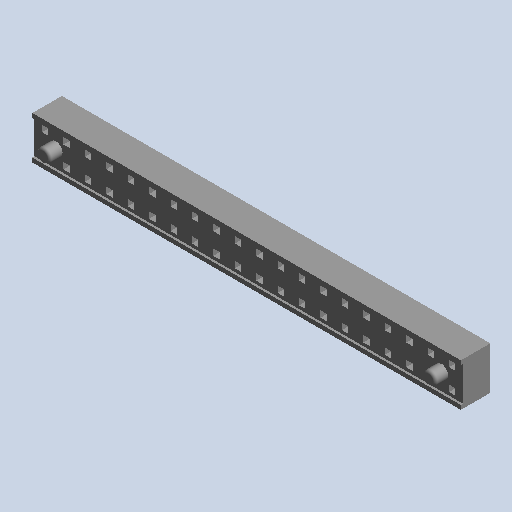
# Autodesk Inventor part: HLE-120-02-DV-A_socket
Saved by Autodesk Inventor 2022 (Build 260153000, 153)
## iProperties
Category: PARTsolutions
Company: SAMTEC
Part Number: HLE-120-02-DV-A_socket
Material: Generic
Catalog Web Link: www.cadenas.de
Description: HLE--Socket
Vendor: SAMTEC
Document SubType Name: Modeling
Designer: partserver
Manufacturer: SAMTEC
Mass: 0.759119 g
Surface Area: 14.3634 cm^2
Volume: 0.759119 cm^3
Density: 1 g/cm^3
Appearance: PSOLRGB-175-175-175
PSOL_IDENT_0: {$CADENAS_DATA\23d-libs\samtec\modelling\hle\parts\hle_socket.prj},196 {VTYP=3D},{NB=HLE-120-02-DV-A
PSOL_IDENT_1: _socket},{LINA=HLE-120-02-DV-A_socket},{NN=HLE-},{DATE=08.04.2016 05:41:54},{GEOMDATE=07.04.2016 12:
PSOL_IDENT_2: 48:00},{VERSION=},{LINEID=10},{WBVAR=POS,AOPT,LCOPT},{WBNUMERIC=}  {NB=HLE-120-02-DV-A_socket},{LINA=
PSOL_IDENT_3: HLE-120-02-DV-A_socket},{KT=DUMMY},{PN=HLE-120-02-DV-A},{SERIES=HLE},{POSALG=  '02' , '-02' , '03' ,
PSOL_IDENT_4: '-03' , '04' , '-04' , '05' , '-05' , '06' , '-06' , '07' , '-07' , '08' , '-08' , '09' , '-09' , '
PSOL_IDENT_5: 10' , '-10' , '11' , '-11' , '12' , '-12' , '13' , '-13' , '14' , '-14' , '15' , '-15' , '16' , '-16'
PSOL_IDENT_6: , '17' , '-17' , '18' , '-18' , '19' , '-19' , '20' , '-20' , '21' , '-21' , '22' , '-22' , '23' , '
PSOL_IDENT_7: -23' , '24' , '-24' , '25' , '-25' , '26' , '-26' , '27' , '-27' , '28' , '-28' , '29' , '-29' , '30'
PSOL_IDENT_8: , '-30' , '31' , '-31' , '32' , '-32' , '33' , '-33' , '34' , '-34' , '35' , '-35' , '36' , '-36' ,
PSOL_IDENT_9: '37' , '-37' , '38' , '-38' , '39' , '-39' , '40' , '-40'  , '41' , '-41' , '42' , '-42' , '43' , '
PSOL_IDENT_10: -43' , '44' , '-44' , '45' , '-45' , '46' , '-46' , '47' , '-47' , '48' , '-48' , '49' , '-49' , '50'
PSOL_IDENT_11: , '-50'   },{POS=20},{LSALG=  '02' , '-02 - Surface Mount'  },{LS=02 - Surface Mount},{ROPTALG=   '
PSOL_IDENT_12: DV' , '-DV - Double Vertical'  },{ROPT=DV},{AOPTALG=    ''  , 'Not Selected'  ,  'A' , '-A - Alignme
PSOL_IDENT_13: nt Pins'   },{AOPT=A},{LCOPTALG= '' , 'Not Available' },{LCOPT=},{B=0.138},{PINS=20},{W=0.2000},{LC=
PSOL_IDENT_14: 0.050},{L=2.00000},{PINW=0.020},{PITCH=0.1000},{PITCH2=0.1000},{AOPTPN=-A},{LCPN=}
NB: HLE-120-02-DV-A_socket
NN: HLE-
NT: Socket
NBSYN: $PN._socket
LINA: HLE-120-02-DV-A_socket
CATALOG: Samtec
PN: HLE-120-02-DV-A
SERIES: HLE
POS: -20
LS: 02 - Surface Mount
ROPT: DV
AOPT: -A - Alignment Pins
LCOPT: Not Available
B: 0.138
W: 0.2
LC: 0.05
L: 2
PINW: 0.02
PITCH: 0.1
PITCH2: 0.1
SUPPLIER: SAMTEC
ARTICLENO: HLE-120-02-DV-A_socket
BOMINFO: HLE-120-02-DV-A_socket
CREATOR: CADENAS GmbH
Title: HLE-120-02-DV-A_socket
Author: Cadenas PARTsolutions
Comments: Socket
Autodesk Inventor part; units mm, degrees
sketch "Sketch_1" plane through (0, 0, 0) normal (0, 1, 0) x (1, 0, 0)
  line L0 (-25.4, 2.54) -> (-25.4, -2.54)
  line L1 (-25.4, -2.54) -> (25.4, -2.54)
  line L2 (25.4, -2.54) -> (25.4, 2.54)
  line L3 (25.4, 2.54) -> (-25.4, 2.54)
  line L4 (23.749, -0.889) -> (23.749, -1.651)
  line L5 (23.749, -1.651) -> (24.511, -1.651)
  line L6 (24.511, -1.651) -> (24.511, -0.889)
  line L7 (24.511, -0.889) -> (23.749, -0.889)
  line L8 (23.749, 1.651) -> (23.749, 0.889)
  line L9 (23.749, 0.889) -> (24.511, 0.889)
  line L10 (24.511, 0.889) -> (24.511, 1.651)
  line L11 (24.511, 1.651) -> (23.749, 1.651)
  line L12 (21.209, -0.889) -> (21.209, -1.651)
  line L13 (21.209, -1.651) -> (21.971, -1.651)
  line L14 (21.971, -1.651) -> (21.971, -0.889)
  line L15 (21.971, -0.889) -> (21.209, -0.889)
  line L16 (21.209, 1.651) -> (21.209, 0.889)
  line L17 (21.209, 0.889) -> (21.971, 0.889)
  line L18 (21.971, 0.889) -> (21.971, 1.651)
  line L19 (21.971, 1.651) -> (21.209, 1.651)
  line L20 (18.669, -0.889) -> (18.669, -1.651)
  line L21 (18.669, -1.651) -> (19.431, -1.651)
  line L22 (19.431, -1.651) -> (19.431, -0.889)
  line L23 (19.431, -0.889) -> (18.669, -0.889)
  line L24 (18.669, 1.651) -> (18.669, 0.889)
  line L25 (18.669, 0.889) -> (19.431, 0.889)
  line L26 (19.431, 0.889) -> (19.431, 1.651)
  line L27 (19.431, 1.651) -> (18.669, 1.651)
  line L28 (16.129, -0.889) -> (16.129, -1.651)
  line L29 (16.129, -1.651) -> (16.891, -1.651)
  line L30 (16.891, -1.651) -> (16.891, -0.889)
  line L31 (16.891, -0.889) -> (16.129, -0.889)
  line L32 (16.129, 1.651) -> (16.129, 0.889)
  line L33 (16.129, 0.889) -> (16.891, 0.889)
  line L34 (16.891, 0.889) -> (16.891, 1.651)
  line L35 (16.891, 1.651) -> (16.129, 1.651)
  line L36 (13.589, -0.889) -> (13.589, -1.651)
  line L37 (13.589, -1.651) -> (14.351, -1.651)
  line L38 (14.351, -1.651) -> (14.351, -0.889)
  line L39 (14.351, -0.889) -> (13.589, -0.889)
  line L40 (13.589, 1.651) -> (13.589, 0.889)
  line L41 (13.589, 0.889) -> (14.351, 0.889)
  line L42 (14.351, 0.889) -> (14.351, 1.651)
  line L43 (14.351, 1.651) -> (13.589, 1.651)
  line L44 (11.049, -0.889) -> (11.049, -1.651)
  line L45 (11.049, -1.651) -> (11.811, -1.651)
  line L46 (11.811, -1.651) -> (11.811, -0.889)
  line L47 (11.811, -0.889) -> (11.049, -0.889)
  line L48 (11.049, 1.651) -> (11.049, 0.889)
  line L49 (11.049, 0.889) -> (11.811, 0.889)
  line L50 (11.811, 0.889) -> (11.811, 1.651)
  line L51 (11.811, 1.651) -> (11.049, 1.651)
  line L52 (8.509, -0.889) -> (8.509, -1.651)
  line L53 (8.509, -1.651) -> (9.271, -1.651)
  line L54 (9.271, -1.651) -> (9.271, -0.889)
  line L55 (9.271, -0.889) -> (8.509, -0.889)
  line L56 (8.509, 1.651) -> (8.509, 0.889)
  line L57 (8.509, 0.889) -> (9.271, 0.889)
  line L58 (9.271, 0.889) -> (9.271, 1.651)
  line L59 (9.271, 1.651) -> (8.509, 1.651)
  line L60 (5.969, -0.889) -> (5.969, -1.651)
  line L61 (5.969, -1.651) -> (6.731, -1.651)
  line L62 (6.731, -1.651) -> (6.731, -0.889)
  line L63 (6.731, -0.889) -> (5.969, -0.889)
  line L64 (5.969, 1.651) -> (5.969, 0.889)
  line L65 (5.969, 0.889) -> (6.731, 0.889)
  line L66 (6.731, 0.889) -> (6.731, 1.651)
  line L67 (6.731, 1.651) -> (5.969, 1.651)
  line L68 (3.429, -0.889) -> (3.429, -1.651)
  line L69 (3.429, -1.651) -> (4.191, -1.651)
  line L70 (4.191, -1.651) -> (4.191, -0.889)
  line L71 (4.191, -0.889) -> (3.429, -0.889)
  line L72 (3.429, 1.651) -> (3.429, 0.889)
  line L73 (3.429, 0.889) -> (4.191, 0.889)
  line L74 (4.191, 0.889) -> (4.191, 1.651)
  line L75 (4.191, 1.651) -> (3.429, 1.651)
  line L76 (0.889, -0.889) -> (0.889, -1.651)
  line L77 (0.889, -1.651) -> (1.651, -1.651)
  line L78 (1.651, -1.651) -> (1.651, -0.889)
  line L79 (1.651, -0.889) -> (0.889, -0.889)
  line L80 (0.889, 1.651) -> (0.889, 0.889)
  line L81 (0.889, 0.889) -> (1.651, 0.889)
  line L82 (1.651, 0.889) -> (1.651, 1.651)
  line L83 (1.651, 1.651) -> (0.889, 1.651)
  line L84 (-1.651, -0.889) -> (-1.651, -1.651)
  line L85 (-1.651, -1.651) -> (-0.889, -1.651)
  line L86 (-0.889, -1.651) -> (-0.889, -0.889)
  line L87 (-0.889, -0.889) -> (-1.651, -0.889)
  line L88 (-1.651, 1.651) -> (-1.651, 0.889)
  line L89 (-1.651, 0.889) -> (-0.889, 0.889)
  line L90 (-0.889, 0.889) -> (-0.889, 1.651)
  line L91 (-0.889, 1.651) -> (-1.651, 1.651)
  line L92 (-4.191, -0.889) -> (-4.191, -1.651)
  line L93 (-4.191, -1.651) -> (-3.429, -1.651)
  line L94 (-3.429, -1.651) -> (-3.429, -0.889)
  line L95 (-3.429, -0.889) -> (-4.191, -0.889)
  line L96 (-4.191, 1.651) -> (-4.191, 0.889)
  line L97 (-4.191, 0.889) -> (-3.429, 0.889)
  line L98 (-3.429, 0.889) -> (-3.429, 1.651)
  line L99 (-3.429, 1.651) -> (-4.191, 1.651)
  line L100 (-6.731, -0.889) -> (-6.731, -1.651)
  line L101 (-6.731, -1.651) -> (-5.969, -1.651)
  line L102 (-5.969, -1.651) -> (-5.969, -0.889)
  line L103 (-5.969, -0.889) -> (-6.731, -0.889)
  line L104 (-6.731, 1.651) -> (-6.731, 0.889)
  line L105 (-6.731, 0.889) -> (-5.969, 0.889)
  line L106 (-5.969, 0.889) -> (-5.969, 1.651)
  line L107 (-5.969, 1.651) -> (-6.731, 1.651)
  line L108 (-9.271, -0.889) -> (-9.271, -1.651)
  line L109 (-9.271, -1.651) -> (-8.509, -1.651)
  line L110 (-8.509, -1.651) -> (-8.509, -0.889)
  line L111 (-8.509, -0.889) -> (-9.271, -0.889)
  line L112 (-9.271, 1.651) -> (-9.271, 0.889)
  line L113 (-9.271, 0.889) -> (-8.509, 0.889)
  line L114 (-8.509, 0.889) -> (-8.509, 1.651)
  line L115 (-8.509, 1.651) -> (-9.271, 1.651)
  line L116 (-11.811, -0.889) -> (-11.811, -1.651)
  line L117 (-11.811, -1.651) -> (-11.049, -1.651)
  line L118 (-11.049, -1.651) -> (-11.049, -0.889)
  line L119 (-11.049, -0.889) -> (-11.811, -0.889)
  line L120 (-11.811, 1.651) -> (-11.811, 0.889)
  line L121 (-11.811, 0.889) -> (-11.049, 0.889)
  line L122 (-11.049, 0.889) -> (-11.049, 1.651)
  line L123 (-11.049, 1.651) -> (-11.811, 1.651)
  line L124 (-14.351, -0.889) -> (-14.351, -1.651)
  line L125 (-14.351, -1.651) -> (-13.589, -1.651)
  line L126 (-13.589, -1.651) -> (-13.589, -0.889)
  line L127 (-13.589, -0.889) -> (-14.351, -0.889)
  line L128 (-14.351, 1.651) -> (-14.351, 0.889)
  line L129 (-14.351, 0.889) -> (-13.589, 0.889)
  line L130 (-13.589, 0.889) -> (-13.589, 1.651)
  line L131 (-13.589, 1.651) -> (-14.351, 1.651)
  line L132 (-16.891, -0.889) -> (-16.891, -1.651)
  line L133 (-16.891, -1.651) -> (-16.129, -1.651)
  line L134 (-16.129, -1.651) -> (-16.129, -0.889)
  line L135 (-16.129, -0.889) -> (-16.891, -0.889)
  line L136 (-16.891, 1.651) -> (-16.891, 0.889)
  line L137 (-16.891, 0.889) -> (-16.129, 0.889)
  line L138 (-16.129, 0.889) -> (-16.129, 1.651)
  line L139 (-16.129, 1.651) -> (-16.891, 1.651)
  line L140 (-19.431, -0.889) -> (-19.431, -1.651)
  line L141 (-19.431, -1.651) -> (-18.669, -1.651)
  line L142 (-18.669, -1.651) -> (-18.669, -0.889)
  line L143 (-18.669, -0.889) -> (-19.431, -0.889)
  line L144 (-19.431, 1.651) -> (-19.431, 0.889)
  line L145 (-19.431, 0.889) -> (-18.669, 0.889)
  line L146 (-18.669, 0.889) -> (-18.669, 1.651)
  line L147 (-18.669, 1.651) -> (-19.431, 1.651)
  line L148 (-21.971, -0.889) -> (-21.971, -1.651)
  line L149 (-21.971, -1.651) -> (-21.209, -1.651)
  line L150 (-21.209, -1.651) -> (-21.209, -0.889)
  line L151 (-21.209, -0.889) -> (-21.971, -0.889)
  line L152 (-21.971, 1.651) -> (-21.971, 0.889)
  line L153 (-21.971, 0.889) -> (-21.209, 0.889)
  line L154 (-21.209, 0.889) -> (-21.209, 1.651)
  line L155 (-21.209, 1.651) -> (-21.971, 1.651)
  line L156 (-24.511, -0.889) -> (-24.511, -1.651)
  line L157 (-24.511, -1.651) -> (-23.749, -1.651)
  line L158 (-23.749, -1.651) -> (-23.749, -0.889)
  line L159 (-23.749, -0.889) -> (-24.511, -0.889)
  line L160 (-24.511, 1.651) -> (-24.511, 0.889)
  line L161 (-24.511, 0.889) -> (-23.749, 0.889)
  line L162 (-23.749, 0.889) -> (-23.749, 1.651)
  line L163 (-23.749, 1.651) -> (-24.511, 1.651)
  constraints: 328 end point
extrude "Extrusion1" add sketch "Sketch_1" along normal blind 3.5052
sketch "Sketch_4" plane through (0, 0, 0) normal (1, 0, 0) x (0, 1, 0)
  line L0 (0.254, 2.032) -> (0, 2.032)
  line L1 (0, 2.032) -> (0, -2.032)
  line L2 (0, -2.032) -> (0.254, -2.032)
  line L3 (0.254, -2.032) -> (0.254, 2.032)
  constraints: 8 end point
extrude "Extrusion2" cut sketch "Sketch_4" along normal mid plane 50.8
sketch "Sketch_9" plane through (0, 0, 0) normal (0, 0, 1) x (1, 0, 0)
  line L0 (22.86, -1.27) -> (22.86, 0.635)
  line L1 (22.86, 0.635) -> (23.6538, 0.635)
  line L2 (23.6538, 0.635) -> (23.6538, -0.9842)
  arc A0 (23.368, -1.27) -> (23.6538, -0.9842) centre (23.368, -0.9843) ccw
  line L3 (23.368, -1.27) -> (22.86, -1.27)
  line L4 (22.86, -1.27) -> (22.86, 0.635)
  constraints: 10 end point, 2 point on circle, 1 centre point
revolve "Revolution1" add sketch "Sketch_9" angle 360 about axis through (22.86, -1.27, 0) along (0, -1, 0)
sketch "Sketch_10" plane through (0, 0, 0) normal (0, 0, 1) x (1, 0, 0)
  line L0 (-22.86, -1.27) -> (-22.86, 0.635)
  line L1 (-22.86, 0.635) -> (-22.0663, 0.635)
  line L2 (-22.0663, 0.635) -> (-22.0663, -0.9525)
  arc A0 (-22.3837, -1.27) -> (-22.0663, -0.9525) centre (-22.3838, -0.9525) ccw
  line L3 (-22.3837, -1.27) -> (-22.86, -1.27)
  line L4 (-22.86, -1.27) -> (-22.86, 0.635)
  constraints: 10 end point, 2 point on circle, 1 centre point
revolve "Revolution2" add sketch "Sketch_10" angle 360 about axis through (-22.86, -1.27, 0) along (0, -1, 0)
sketch "Sketch_11" plane through (0, 3.5052, 0) normal (0, 1, 0) x (1, 0, 0)
  line L0 (-23.0505, 1.27) -> (-23.0505, -1.27)
  line L1 (-23.0505, -1.27) -> (-22.6695, -1.27)
  line L2 (-22.6695, -1.27) -> (-22.6695, 1.27)
  line L3 (-22.6695, 1.27) -> (-23.0505, 1.27)
  constraints: 8 end point
extrude "Extrusion3" cut sketch "Sketch_11" against normal blind 1.27
pattern_linear "Rectangular Pattern1" count 19 spacing 2.54 along (1, 0, 0) of "Extrusion3"
ref_plane "socket_to_dummy_XY" through (0, 0, 0) normal (0, -1, 0) x (1, 0, 0)
ref_plane "socket_to_dummy_YZ" through (0, 0, 0) normal (1, 0, 0) x (0, 0, 1)
ref_plane "socket_to_dummy_ZX" through (0, 0, 0) normal (0, 0, 1) x (0, -1, 0)
ref_plane "socket_to_pad_XY" through (0, 3.5052, 0) normal (0, 1, 0) x (1, 0, 0)
ref_plane "socket_to_pad_YZ" through (0, 3.5052, 0) normal (1, 0, 0) x (0, 0, -1)
ref_plane "socket_to_pad_ZX" through (0, 3.5052, 0) normal (0, 0, -1) x (0, 1, 0)
body "Solid1"
